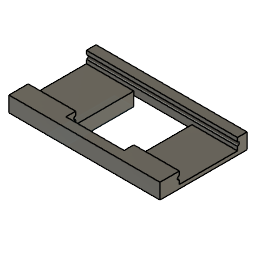
基板設置個所 v4 (Autodesk Fusion 360 design; units mm, degrees)
Autodesk Fusion 360 part; units mm, degrees
sketch "スケッチ1" plane through (0, 0, 0) normal (0, 0, 1) x (1, 0, 0)
  line L0 (0, 0) -> (-50, 0)
  line L1 (-50, 0) -> (-50, -35)
  line L2 (-50, -35) -> (0, -35)
  line L3 (0, -35) -> (0, 0)
  line L4 (-65, 5) -> (15, 5)
  line L5 (15, 5) -> (15, -40)
  line L6 (15, -40) -> (-65, -40)
  line L7 (-65, -40) -> (-65, 5)
  constraint horizontal L0
  constraint vertical L1
  constraint horizontal L2
  constraint vertical L3
  constraint coincident L0.start L3.end
  constraint horizontal L4
  constraint vertical L5
  constraint horizontal L6
  constraint vertical L7
extrude "押し出し1" add sketch "スケッチ1" against normal blind 5 contours L0 L1 L2 L3
extrude "押し出し2" add sketch "スケッチ1" along normal blind 5 contours L0 L1 L2 L3 | L4 L5 L6 L7
sketch "スケッチ2" plane through (0, 0, 5) normal (0, 0, 1) x (-1, 0, 0)
  line L0 (65, 40) -> (-15, 40)
  line L1 (-15, 40) -> (-15, -5)
  line L2 (-15, -5) -> (65, -5)
  line L3 (65, -5) -> (65, 40)
  line L4 (-15, 0) -> (65, 0)
  line L5 (65, 0) -> (65, 30)
  line L6 (65, 30) -> (-15, 30)
  line L7 (-15, 30) -> (-15, 0)
  constraint horizontal L4
  constraint vertical L5
  constraint horizontal L6
  constraint vertical L7
  constraint coincident L3 L5.end
  constraint coincident L1 L4.start
extrude "押し出し3" cut sketch "スケッチ2" against normal blind 3 contours L1 L3 L4 L5 L6 L7
sketch "スケッチ3" plane through (0, 0, -5) normal (0, 0, -1) x (1, 0, 0)
  line L0 (0, 0) -> (0, 35)
  line L1 (0, 35) -> (-50, 35)
  line L2 (-50, 35) -> (-50, 0)
  line L3 (-50, 0) -> (0, 0)
  line L4 (-10, 0) -> (-40, 0)
  line L5 (-40, 0) -> (-40, 35)
  line L6 (-40, 35) -> (-10, 35)
  line L7 (-10, 35) -> (-10, 0)
  constraint horizontal L4
  constraint vertical L5
  constraint horizontal L6
  constraint vertical L7
  constraint coincident L1 L5.end
  constraint coincident L3 L4.start
extrude "押し出し4" cut sketch "スケッチ3" against normal blind 10 contours L1 L3 L4 L5 L6 L7
extrude "押し出し5" add 2 faces at (-38.3333, 3.3333, 5) (-56.6667, -35, 5) along direction (0, 0, 1) blind 3
sketch "スケッチ4" plane through (-65, 0, 0) normal (-1, 0, 0) x (0, -1, 0)
  line L0 (0, 2) -> (0, 8)
  line L1 (0, 8) -> (-5, 8)
  line L2 (-5, 8) -> (-5, 0)
  line L3 (-5, 0) -> (40, 0)
  line L4 (40, 0) -> (40, 8)
  line L5 (40, 8) -> (30, 8)
  line L6 (30, 8) -> (30, 2)
  line L7 (30, 2) -> (0, 2)
  line L8 (0, 5) -> (30, 5)
  line L9 (0, 4) -> (30, 4)
  arc A0 (30, 4) -> (30, 6) centre (30, 5) ccw
  line L10 (30, 6) -> (0, 6)
  arc A1 (0, 6) -> (0, 4) centre (0, 5) ccw
  line L11 (0, 5) -> (30, 5) construction
  constraint midpoint L0 L8.start
  constraint midpoint L6 L8.end
  constraint tangent L9 A0
  constraint tangent A0 L10
  constraint parallel L9 L10
  constraint tangent L10 A1
  constraint tangent L9 A1
  constraint coincident L8.end A0.centre
  constraint perpendicular L6 L11
  constraint coincident L8.start A1.centre
extrude "押し出し6" cut sketch "スケッチ4" against normal blind 80 contours L0 A1 | L6 A0
sketch "スケッチ5" plane through (0, 0, -5) normal (0, 0, -1) x (1, 0, 0)
  line L0 (-40, 0) -> (-40, 35)
  line L1 (-40, 35) -> (-50, 35)
  line L2 (-50, 35) -> (-50, 0)
  line L3 (-50, 0) -> (-40, 0)
extrude "押し出し7" cut 1 faces at (-65, -36.9916, 4.2592) along direction (1, 0, 0) blind 1
extrude "押し出し8" cut 1 faces at (-64, -36.9916, 4.2592) along direction (1, 0, 0) blind 1
extrude "押し出し9" cut 1 faces at (15, -36.9916, 4.2592) along direction (-1, 0, 0) blind 1
extrude "押し出し10" add 1 faces at (-63, -36.9916, 4.2592) along direction (-1, 0, 0) blind 0.5
extrude "押し出し11" cut 1 faces at (14, -36.9916, 4.2592) along direction (-1, 0, 0) blind 0.5
extrude "押し出し12" cut 1 faces at (0, -23.3333, -3.3333) along direction (-1, 0, 0) blind 0.25
extrude "押し出し13" cut 1 faces at (-50, -11.6667, -3.3333) along direction (1, 0, 0) blind 0.25
extrude "押し出し14" add 1 faces at (-63.5, -36.9916, 4.2592) along direction (-1, 0, 0) blind 1
